Bearing (Autodesk Fusion 360 design; units mm, degrees)
Autodesk Fusion 360 part; units mm, degrees
note: some values were not read from the file. Set by a fixed rule: which sketch regions a step uses.
sketch "Sketch1" plane through (0, 0, 0) normal (0, 1, 0) x (1, 0, 0)
  line L0 (2, -4.25) -> (-2, -4.25)
  line L1 (-2, -4.25) -> (-2, -5)
  line L2 (-2, -5) -> (2, -5)
  line L3 (2, -5) -> (2, -4.25)
  line L4 (2, -4.25) -> (-2, -5) construction
  line L5 (-2, -4.25) -> (2, -5) construction
  line L6 (2, -2.5) -> (-2, -2.5)
  line L7 (-2, -2.5) -> (-2, -3.15)
  line L8 (-2, -3.15) -> (2, -3.15)
  line L9 (2, -3.15) -> (2, -2.5)
  line L10 (2, -2.5) -> (-2, -3.15) construction
  line L11 (-2, -2.5) -> (2, -3.15) construction
  circle A0 centre (0, -3.7) radius 0.75
  line L12 (0, -4.45) -> (0, -2.95)
  point P0 (0, -4.625)
  point P1 (0, -2.825)
  dimension "d1" = 4
  dimension "d2" = 0.75
  dimension "d3" = 4
  dimension "d4" = 0.65
  dimension "d5" = 2.5
  dimension "d6" = 2.5
  dimension "d7" = 1.5
  constraint horizontal L0
  constraint perpendicular L0 L1
  constraint parallel L0 L2
  constraint parallel L1 L3
  constraint coincident L4 P0
  constraint coincident L5 P0
  constraint horizontal L6
  constraint perpendicular L6 L7
  constraint parallel L6 L8
  constraint parallel L7 L9
  constraint coincident L10 P1
  constraint coincident L11 P1
  constraint coincident A0 L12.start
  constraint coincident A0 L12.end
  constraint vertical L12
  measures "d1" distance of L1.end L2.end
  measures "d2" distance of L0.end L1.end
  measures "d3" distance of L7.end L8.end
  measures "d4" distance of L6.end L7.end
  measures "d5" distance of L2.end L6.start
  measures "d6" distance of origin L6
  measures "d7" diameter of A0
revolve "Revolve1" add sketch "Sketch1" angle 360 about axis through (1.75, 0, 0) along (1, 0, 0) contours L0 L1 L2 L3 A0 | L6 L7 L8 L9 A0 makes body 1 at (-0.6667, 0.2492, 4.9938) makes body 2 at (0.6667, 0.1246, 2.4969)
revolve "Revolve2" add sketch "Sketch1" angle 360 about axis through (0, 0, 1.75) along (0, 0, 1) separate body contours L0 A0 L12 | L0 L8 A0 L12 | L8 A0 L12 picked at (0.0372, -4.3805) picked at (0.25, -3.7) picked at (0.0372, -3.0195) makes body 3
pattern_circular "C-Pattern1" count 6 over 360 about axis through (1.75, 0, 0) along (1, 0, 0) of bodies 3 makes body 4 at (0.3715, -3.6148, 1.3441) makes body 5 at (0.3715, -2.9714, -2.4585) makes body 6 at (0.3715, 0.6434, -3.8026) makes body 7 at (-0.3715, 3.6148, -1.3441) makes body 8 at (0.3715, 2.9714, 2.4585)
fillet "Fillet1" radius 0.1 8 edges at (2, -1.8081, -4.6616) (-2, -1.8081, -4.6616) (-2, -1.5369, -3.9624) (2, -1.5369, -3.9624) (2, -1.1391, -2.9368) (2, -0.904, -2.3308) (-2, -1.1391, -2.9368) (-2, -0.904, -2.3308) on bodies 1 2
sketch "Sketch2" plane through (0, 0, 0) normal (1, 0, 0) x (0, 1, 0)
  circle A0 centre (0, 0) radius 3.55
  circle A1 centre (0, 0) radius 3.85
  dimension "d16" = 7.1
  dimension "d17" = 7.7
  constraint coincident A0.centre A1.centre
  measures "d16" diameter of A0
  measures "d17" diameter of A1
extrude "Extrude1" add sketch "Sketch2" along normal blind 1.2 separate body makes body 9
combine "Combine1" operation cut target body 9 tool bodies 3 8 4 5 6 7 keep tools
shell "Shell1" thickness 0.1 removed faces 3 at (1.2, 3.7224, -0.3676) at (0.5175, 2.6431, -2.7994) at (0.515, 1.0316, 3.3968) on bodies 9
mirror "Mirror1" about plane through (0, 0, 0) normal (1, 0, 0) of bodies 9 merged
